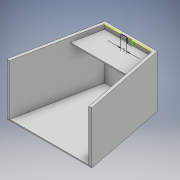
# Autodesk Inventor part: Modulo
Saved by Autodesk Inventor 2017 (Build 210142000, 142)
## iProperties
Created: 2016-07-03
Part Number: Modulo
Material: Generic
Document SubType Name: Modeling
Designer: Ing
Density: 1 g/cm^3
Appearance: Default
Author: Ing
Autodesk Inventor part; units mm, degrees
ref_plane "YZ Plane" through (0, 0, 0) normal (1, 0, 0) x (0, 1, 0)
ref_plane "XZ Plane" through (0, 0, 0) normal (0, 1, 0) x (-1, 0, 0)
ref_plane "XY Plane" through (0, 0, 0) normal (0, 0, 1) x (1, 0, 0)
sketch "Sketch1" plane through (0, 0, 0) normal (0, 0, 1) x (1, 0, 0)
  point P0 (0, 0)
sketch "Sketch2" plane through (0, 0, 0) normal (0, 0, 1) x (1, 0, 0)
  line L0 (0, 0) -> (-21, 0)
  line L1 (0, 0) -> (21, 0)
  line L2 (21, -70) -> (-21, -70)
  line L3 (-21, -70) -> (-35, -70)
  line L4 (-35, -70) -> (-21, 0)
  line L5 (21, -70) -> (35, -70)
  line L6 (35, -70) -> (21, 0)
  line L7 (-35, -70) -> (-37.4515, -69.5097)
  line L8 (-23.4515, 0.4903) -> (-37.4515, -69.5097)
  line L9 (-23.4515, 0.4903) -> (-23.0495, 2.5)
  line L10 (35, -70) -> (37.4515, -69.5097)
  line L11 (23.4515, 0.4903) -> (37.4515, -69.5097)
  line L12 (-23.0495, 2.5) -> (23.0495, 2.5)
  line L13 (23.0495, 2.5) -> (23.4515, 0.4903)
  dimension "d3" = 21
  dimension "d4" = 21
  dimension "d5" = 70
  dimension "d6" = 14
  dimension "d7" = 14
  constraints: 28 end point, 4 horizontal, 3 point on line, 1 collinear, 1 parallel
  measures "d3" distance of L0.start L0.end
  measures "d4" distance of L0.start L1.end
  measures "d5" distance of L1.end L2.start
  measures "d6" distance of L2.end L3.end
  measures "d7" distance of L2.start L5.end
extrude "Extrusion1" add sketch "Sketch2" along normal blind 45 contours L0 L4 L7 L8 L9 L12 L13 L11 L10 L6 L1
sketch "Sketch3" plane through (-21, 0, 0) normal (0, -1, 0) x (1, 0, 0)
  point P0 (21, 0)
sketch "Sketch5" plane through (-21, 0, 0) normal (0, -1, 0) x (1, 0, 0)
  line L0 (0, 45) -> (42, 45) projected
  line L1 (19.4909, 45) -> (14.4909, 45)
  line L2 (24.3761, 45) -> (24.3761, 40)
  line L3 (24.3761, 40) -> (42, 40)
  line L4 (42, 40) -> (0, 40)
  point P0 (21, 0)
  dimension "d16" = 5
  dimension "d17" = 5
  constraints: 8 end point, 4 point on line, 2 perpendicular
  measures "d16" distance of L1.start L1.end
  measures "d17" distance of L2.start L2.end
sketch "Sketch6" plane through (-21, 0, 0) normal (0, -1, 0) x (1, 0, 0)
  point P0 (21, 0)
ref_plane "Work Plane6" through (21, 0, 40) normal (0, 0, -1) x (-1, 0, 0)
sketch "Sketch7" plane through (21, 0, 40) normal (0, 0, -1) x (-1, 0, 0)
  line L0 (42, 0) -> (0, 0) projected
  line L1 (0, 0) -> (42, 0)
  line L2 (42, -25) -> (47, -25)
  line L3 (56, -70) -> (42, 0) projected
  line L4 (42, -25) -> (-5, -25)
  line L5 (0, 0) -> (-14, -70) projected
  line L6 (0, 0) -> (-5, -25)
  line L7 (47, -25) -> (42, 0)
  line L8 (44.0495, 2.5) -> (58.4515, -69.5097) projected
  line L9 (47, -25) -> (42, -25)
  point P0 (21, 0)
  dimension "d19" = 25
  constraints: 12 end point, 3 collinear, 3 point on line, 1 parallel
  measures "d19" distance of L0.start L2.start
extrude "Extrusion3" add sketch "Sketch7" against normal blind 1
sketch "Sketch8" plane through (0, 0, 0) normal (0, 0, -1) x (-1, 0, 0)
  point P0 (0, 0)
sketch "Sketch9" plane through (0, 0, 0) normal (0, 0, -1) x (-1, 0, 0)
  line L0 (-37.4515, -69.5097) -> (-23.0495, 2.5) projected
  line L1 (37.4515, -69.5097) -> (-37.4515, -69.5097)
  line L2 (-37.4515, -69.5097) -> (-23.0495, 2.5)
  line L3 (-23.0495, 2.5) -> (23.0495, 2.5)
  line L4 (23.0495, 2.5) -> (37.4515, -69.5097) projected
  line L5 (23.0495, 2.5) -> (37.4515, -69.5097)
  line L6 (23.0495, 2.5) -> (37.4515, -69.5097) projected
  line L7 (37.4515, -69.5097) -> (37.4515, -69.5097)
  point P0 (0, 0)
  constraints: 10 end point, 2 collinear, 1 horizontal, 1 parallel, 1 perpendicular
extrude "Extrusion4" add sketch "Sketch9" along normal blind 1
body "Solid1"
